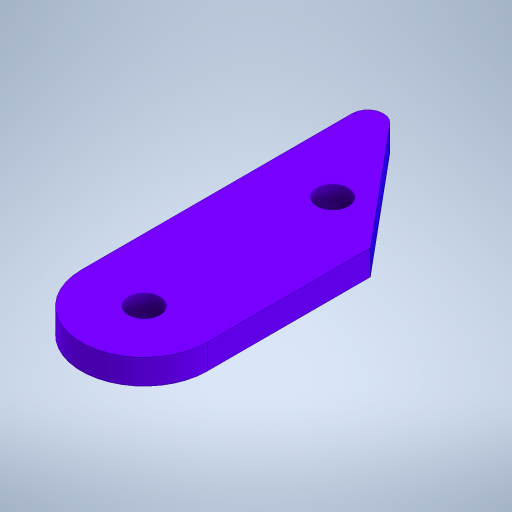
# Autodesk Inventor part: Finger
Saved by Autodesk Inventor 2023.1 (Build 271208000, 208)
## iProperties
Created: 2022-11-06
Part Number: Finger
Material: Generic
Document SubType Name: Modeling
Designer: shubh
Density: 1 g/cm^3
Appearance: Default(3)
Author: shubh
Autodesk Inventor part; units mm, degrees
ref_plane "YZ Plane" through (0, 0, 0) normal (1, 0, 0) x (0, 1, 0)
ref_plane "XZ Plane" through (0, 0, 0) normal (0, 1, 0) x (-1, 0, 0)
ref_plane "XY Plane" through (0, 0, 0) normal (0, 0, 1) x (1, 0, 0)
sketch "Sketch1" plane through (0, 0, 0) normal (0, 1, 0) x (-1, 0, 0)
  line L0 (0, 0) -> (-25.4, 0)
  line L1 (-25.4, 0) -> (-25.4, -45.72)
  line L2 (0, -76.2) -> (0, 0)
  line L3 (-25.4, 0) -> (-25.4, -45.72)
  line L4 (-25.4, -45.72) -> (0, -76.2)
  point P0 (0, -76.2)
  dimension "d2" = 45.72
  dimension "d22" = 25.4
  dimension "d23" = 76.2
  constraints: 10 end point, 1 horizontal, 1 parallel, 1 perpendicular
  measures "d2" distance of L1.end L0.end
  measures "d22" distance of L0.start L0.end
  measures "d23" distance of L2.start L0.start
extrude "Extrusion1" add sketch "Sketch1" along normal blind 5.08
fillet "Fillet2" radius 12.7 1 edges at (25.4, 2.54, 0)
fillet "Fillet3" radius 12.7 1 edges at (0, 2.54, 0)
sketch "Sketch2" plane through (0, 5.08, 0) normal (0, 1, 0) x (1, 0, 0)
  circle A0 centre (12.7, 12.7) radius 3.175
  circle A1 centre (12.7, 50.8) radius 3.175
  point P0 (0, 0)
  dimension "d9" = 6.35
  dimension "d10" = 12.7
  dimension "d11" = 12.7
  dimension "d16" = 6.35
  dimension "d17" = 38.1
  dimension "d18" = 12.7
  constraints: 2 centre point
  measures "d9" diameter of A0
  measures "d10" horizontal distance of point (0, 0) A0.centre
  measures "d11" horizontal distance of point (0, 0) A0.centre
  measures "d16" diameter of A1
  measures "d17" distance of A0.centre A1.centre
  measures "d18" horizontal distance of point (0, 0) A1.centre
extrude "Extrusion2" cut sketch "Sketch2" against normal blind 12.7
fillet "Fillet6" radius 3.175 1 edges at (0, 2.54, -76.2)
body "Solid1"
